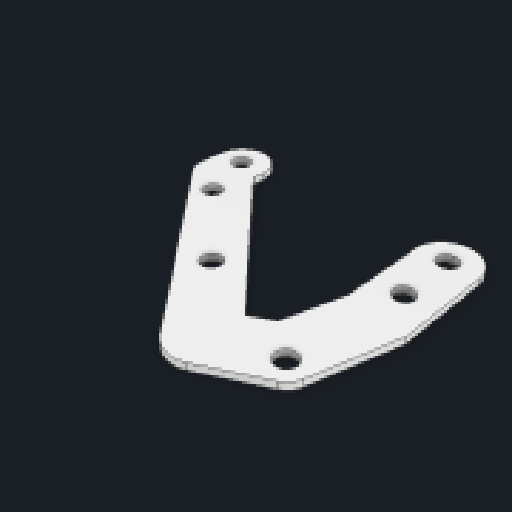
# Autodesk Inventor part: Ring Funnel
Saved by Autodesk Inventor 2025.1 (Build 291241000, 241)
## iProperties
Created: 2024-12-17
Part Number: Ring Funnel
Material: Acetal Resin, White
Document SubType Name: Modeling
Designer: Averey Ku
Density: 1.425 g/cm^3
Appearance: Smooth - White
d0: 0.172 in
d1: 135.00 deg
d2: 0.500 in
d3: 0.250 in
d4: 0.500 in
d5: 0.172 in
d6: 0.172 in
d9: 0.188 in
d10: 1.875 in
d11: 1.469 in
Author: Averey Ku
Autodesk Inventor part; units mm, degrees
ref_plane "YZ Plane" through (0, 0, 0) normal (1, 0, 0) x (0, 1, 0)
ref_plane "XZ Plane" through (0, 0, 0) normal (0, 1, 0) x (-1, 0, 0)
ref_plane "XY Plane" through (0, 0, 0) normal (0, 0, 1) x (1, 0, 0)
sketch "main" plane through (0, 0, 0) normal (0, 0, 1) x (1, 0, 0)
  circle A0 centre (13.3958, 31.4064) radius 2.1844
  line L0 (25.3837, 29.1351) -> (22.5582, 29.1351)
  line L1 (25.3837, 29.1351) -> (25.3095, 29.1351)
  line L2 (20.0497, 41.8351) -> (13.668, 35.4534) construction
  arc A1 (20.0497, 41.8351) -> (15.6723, 40.0972) centre (20.0497, 35.4534) ccw
  circle A2 centre (25.3837, 35.4851) radius 2.1844
  line L3 (25.3837, 41.8351) -> (20.0497, 41.8351)
  line L4 (20.0497, 41.8351) -> (29.0749, 41.8351) construction
  arc A3 (25.3837, 29.1351) -> (25.3837, 41.8351) centre (25.3837, 35.4851) ccw
  circle A4 centre (12.6837, -15.3149) radius 2.1844
  circle A5 centre (-11.9225, -12.1399) radius 2.1844
  arc A6 (-16.0947, -14.4365) -> (-13.1988, -16.7282) centre (-11.9225, -12.1399) ccw
  line L5 (-9.1363, -0.7415) -> (-6.5789, -5.3874)
  line L6 (-22.634, -2.5568) -> (-16.0947, -14.4365)
  line L7 (-6.5789, -5.3874) -> (6.2826, -8.9649)
  line L8 (6.2826, -8.9649) -> (25.3837, -8.9649)
  circle A7 centre (25.3837, -15.3149) radius 2.1844
  arc A8 (25.3837, -21.6649) -> (25.3837, -8.9649) centre (25.3837, -15.3149) ccw
  line L9 (4.5492, -21.6649) -> (25.3837, -21.6649)
  line L10 (4.5492, -21.6649) -> (-13.1988, -16.7282)
  line L11 (22.5582, 29.1351) -> (-9.1363, -0.7415)
  line L12 (-21.4268, 5.126) -> (15.6723, 40.0972)
  circle A9 centre (-3.0276, 13.7434) radius 2.1844
  arc A10 (-21.4268, 5.126) -> (-22.634, -2.5568) centre (-17.0712, 0.5054) ccw
  point P0 (7.4272, 10.3782)
  point P1 (19.0337, 40.8191)
  point P2 (-25.006, 1.7522)
  point P3 (-30.1788, -11.3461)
  dimension "d0" = 4.3688
  dimension "d1" = 135
  dimension "d2" = 12.7
  dimension "d3" = 6.35
  dimension "d4" = 12.7
  dimension "d5" = 4.3688
  dimension "d6" = 4.3688
  dimension "d9" = 4.7625
  dimension "d10" = 47.625
  dimension "d11" = 37.3062
  measures "d0" diameter of A5
  measures "d1" angle of L2 L4
  measures "d2" diameter of A8
  measures "d3" radius of A10
  measures "d4" distance between parallel lines of L12 L11
  measures "d5" diameter of A9
  measures "d6" diameter of A0
  measures "d9" radius of A6
  measures "d10" vertical distance of A5.centre A2.centre
  measures "d11" horizontal distance of A5.centre A2.centre
sketch "Sketch1" plane through (0, 0, 0) normal (0, 1, 0) x (-1, 0, 0)
  circle A0 centre (-4.0925, 11.9832) radius 2.1844
  line L0 (-6.35, -0.0073) -> (-6.3532, 2.8182)
  line L1 (-6.35, -0.0073) -> (-6.3501, 0.0669)
  line L2 (6.3439, 5.3413) -> (-0.0452, 11.7157) construction
  arc A1 (6.3439, 5.3413) -> (4.6009, 9.7167) centre (-0.0379, 5.334) ccw
  circle A2 centre (0, 0) radius 2.1844
  line L3 (6.35, 0.0073) -> (6.3439, 5.3413)
  line L4 (6.3439, 5.3413) -> (6.3542, -3.6839) construction
  arc A3 (-6.35, -0.0073) -> (6.35, 0.0073) centre (0, 0) ccw
  circle A4 centre (-50.8145, 12.6417) radius 2.1844
  circle A5 centre (-47.6678, 37.2516) radius 2.1844
  arc A6 (-49.9692, 41.4211) -> (-52.2575, 38.5226) centre (-47.6678, 37.2516) ccw
  line L5 (-36.2662, 34.4785) -> (-40.9092, 31.9157)
  line L6 (-38.097, 47.9741) -> (-49.9692, 41.4211)
  line L7 (-40.9092, 31.9157) -> (-44.4719, 19.0501)
  line L8 (-44.4719, 19.0501) -> (-44.45, -0.051)
  circle A7 centre (-50.8, -0.0583) radius 2.1844
  arc A8 (-57.15, -0.0656) -> (-44.45, -0.051) centre (-50.8, -0.0583) ccw
  line L9 (-57.1739, 20.769) -> (-57.15, -0.0656)
  line L10 (-57.1739, 20.769) -> (-52.2575, 38.5226)
  line L11 (-6.3532, 2.8182) -> (-36.2662, 34.4785)
  line L12 (-30.4128, 46.7757) -> (4.6009, 9.7167)
  circle A9 centre (-21.7743, 28.3864) radius 2.1844
  arc A10 (-30.4128, 46.7757) -> (-38.097, 47.9741) centre (-35.0285, 42.4147) ccw
  point P0 (0, 0)
  point P1 (-6.3501, 0.0669)
  constraints: 1 other
extrude "Extrusion1" add sketch "Sketch1" along normal blind 1.5875
body "Solid1"
